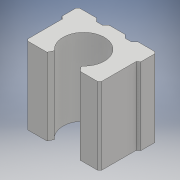
# Autodesk Inventor part: PilowBlockAberto
Saved by Autodesk Inventor 2018 (Build 220112000, 112)
## iProperties
Created: 2018-07-23
Part Number: PilowBlockAberto
Material: Genérico
Document SubType Name: Modeling
Designer: Usuario
Density: 1 g/cm^3
Appearance: Padrão
Mass: 25.4748 g
Surface Area: 89.1124 cm^2
Volume: 25.4748 cm^3
Author: Usuario
Autodesk Inventor part; units mm, degrees
ref_plane "YZ Plane" through (0, 0, 0) normal (1, 0, 0) x (0, 1, 0)
ref_plane "XZ Plane" through (0, 0, 0) normal (0, 1, 0) x (-1, 0, 0)
ref_plane "XY Plane" through (0, 0, 0) normal (0, 0, 1) x (1, 0, 0)
sketch "Esboço1" plane through (0, 0, 0) normal (0, 0, 1) x (1, 0, 0)
  arc A0 (19.1365, -5.3084) -> (5.6379, -5.3084) centre (12.3872, 2.735) ccw
  line L0 (12.3872, 2.735) -> (12.3872, 19.735) construction
  line L1 (32.3872, 18.735) -> (32.3872, 11.735)
  line L2 (-7.6128, 11.735) -> (-7.6128, 18.735)
  circle A1 centre (12.3872, 2.735) radius 4.25 construction
  line L3 (30.0707, -7.865) -> (21.2817, -7.865)
  line L4 (4.3872, -7.865) -> (-5.2963, -7.865)
  line L5 (5.6379, -5.3084) -> (4.3872, -7.865)
  line L6 (19.1365, -5.3084) -> (21.2817, -7.865)
  line L7 (-7.6128, 11.735) -> (-6.2963, 10.6304)
  line L8 (-6.2963, 10.6304) -> (-6.2963, -6.865)
  line L9 (-1.6128, -7.865) -> (-1.6128, 19.735) construction
  line L10 (26.3872, -7.865) -> (26.3872, 19.735) construction
  line L11 (12.3872, 19.735) -> (12.3872, -10.9717) construction
  line L12 (32.3872, 11.735) -> (31.0707, 10.6304)
  line L13 (31.0707, 10.6304) -> (31.0707, -6.865)
  line L14 (1.3434, 19.735) -> (5.648, 19.735) construction
  line L15 (1.8977, 19.735) -> (3.5675, 18.0653)
  line L16 (0.2217, 19.735) -> (2.5831, 19.735) construction
  line L17 (3.5675, 18.0653) -> (6.6886, 18.0653)
  line L18 (6.6886, 18.0653) -> (8.3584, 19.735)
  line L19 (22.8767, 19.735) -> (21.2069, 18.0653)
  line L20 (21.2069, 18.0653) -> (18.0858, 18.0653)
  line L21 (18.0858, 18.0653) -> (16.416, 19.735)
  line L22 (-6.6128, 19.735) -> (1.8977, 19.735)
  line L23 (8.3584, 19.735) -> (16.416, 19.735)
  line L24 (22.8767, 19.735) -> (31.3872, 19.735)
  line L25 (-7.6128, 18.735) -> (-6.6128, 19.735)
  line L26 (-6.2963, -6.865) -> (-5.2963, -7.865)
  line L27 (30.0707, -7.865) -> (31.0707, -6.865)
  line L28 (32.3872, 18.735) -> (31.3872, 19.735)
  point P0 (0, 0)
  point P1 (-7.6128, 19.735)
  point P2 (32.3872, 19.735)
  point P3 (-6.2963, -7.865)
  point P4 (31.0707, -7.865)
  dimension "d0" = 17
  dimension "d2" = 40
  dimension "d4" = 8.5
  dimension "d6" = 20
  dimension "d10" = 8
  dimension "d12" = 14
  dimension "d13" = 14
  dimension "d19" = 1
  dimension "d20" = 1
  dimension "d21" = 1
  dimension "d22" = 1
  dimension "d23" = 1
  dimension "d24" = 1
  dimension "d25" = 1
  dimension "d26" = 1
  constraints: 58 end point, 14 point on line, 11 perpendicular, 7 symmetric about line, 6 horizontal, 6 parallel, 2 centre point, 2 point on circle, 1 coincident, 1 equal length, 1 vertical
  measures "d0" distance of L0.start L0.end
  measures "d2" distance of point (-7.613, 19.735) point (32.387, 19.735)
  measures "d4" diameter of A1
  measures "d6" distance from line of L2 L0.start
  measures "d10" distance of L2.start point (-7.613, 19.735)
  measures "d12" distance from line of L9 L0.start
  measures "d13" distance from line of L10 L0.start
  measures "d19" distance of L2.end point (-7.613, 19.735)
  measures "d20" distance of L22.start point (-7.613, 19.735)
  measures "d21" distance of L8.end point (-6.296, -7.865)
  measures "d22" distance of L4.end point (-6.296, -7.865)
  measures "d23" distance of L3.start point (31.071, -7.865)
  measures "d24" distance of L13.end point (31.071, -7.865)
  measures "d25" distance of L1.start point (32.387, 19.735)
  measures "d26" distance of L24.end point (32.387, 19.735)
extrude "Extrusão1" add sketch "Esboço1" against normal blind 39
sketch "Esboço2" plane through (-6.6128, 19.735, 0) normal (0, 1, 0) x (1, 0, 0)
  line L0 (-1, 0) -> (0.3165, 0)
  line L1 (39, 0) -> (39, 39)
  line L2 (-1, 0) -> (39, 0)
  line L3 (39, 0) -> (39, 39)
  line L4 (39, 39) -> (-1, 39)
  line L5 (-1, 0) -> (-1, 39)
  line L6 (-1, 39) -> (-1, 0)
  line L7 (8.5105, 0) -> (0, 0)
  line L8 (11, 39) -> (1.3165, 39)
  line L9 (27.8945, 0) -> (36.6835, 0)
  line L10 (33, 0) -> (33, 39) construction
  line L11 (29.5, 0) -> (8.5, 0)
  line L12 (19, 0) -> (19, 39) construction
  line L13 (8.5, 39) -> (29.5, 39)
  line L14 (11, 39) -> (1.3165, 39) projected
  line L15 (5, 39) -> (5, 0) construction
  line L16 (1.3165, 0) -> (11, 0) projected
  line L17 (-4.598, 19.5) -> (42.402, 19.5) construction
  line L18 (-10.187, 32.5) -> (53.6518, 32.5) construction
  line L19 (-10.187, 6.5) -> (53.6518, 6.5) construction
  circle A0 centre (5, 32.5) radius 1.6801 construction
  circle A1 centre (33, 32.5) radius 1.5751 construction
  circle A2 centre (5, 6.5) radius 1.6801 construction
  circle A3 centre (33, 6.5) radius 1.5751 construction
  point P0 (6.6128, 0)
  point P1 (12.2507, 0)
  point P2 (25.7493, 0)
  point P3 (25.7493, 39)
  point P4 (12.2507, 39)
  dimension "d29" = 14
  dimension "d31" = 14
  dimension "d32" = 47
  dimension "d33" = 13
  dimension "d34" = 13
  constraints: 32 end point, 11 point on line, 4 centre point, 4 horizontal, 2 midpoint, 2 vertical, 7 other
  measures "d29" distance between parallel lines of L12 L10
  measures "d31" distance between parallel lines of L15 L12
  measures "d32" distance of L17.start L17.end
  measures "d33" distance between parallel lines of L19 L17
  measures "d34" distance between parallel lines of L17 L18
hole "Furo1" at (-1.6128, 19.735, -32.5) at (26.3872, 19.735, -32.5) at (26.3872, 19.735, -6.5) at (-1.6128, 19.735, -6.5) direction (0, -1, 0) diameter 4.134 depth 14.2 tip angle 118 thread size "M5x0.8" class "6H" standard "ANSI Metric M Profile"
equation "\"d20\" = d19"
equation "\"d21\" = d19"
equation "\"d22\" = d21"
equation "\"d23\" = d19"
equation "\"d24\" = d23"
equation "\"d25\" = d19"
equation "\"d26\" = d25"
